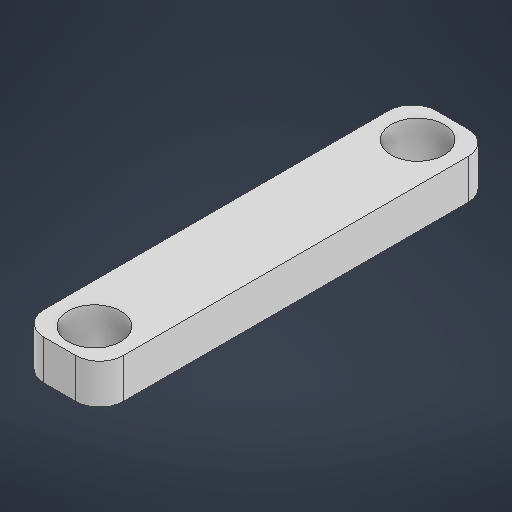
# Autodesk Inventor part: LegLverr
Saved by Autodesk Inventor 2026.2 (Build 302298010, 298A)
## iProperties
Created: 2026-05-06
Part Number: LegLverr
Material: Generic
Document SubType Name: Modeling
Designer: Martina
Density: 1 g/cm^3
Appearance: Default
Author: Martina
Autodesk Inventor part; units mm, degrees
ref_plane "YZ Plane" through (0, 0, 0) normal (1, 0, 0) x (0, 1, 0)
ref_plane "XZ Plane" through (0, 0, 0) normal (0, 1, 0) x (-1, 0, 0)
ref_plane "XY Plane" through (0, 0, 0) normal (0, 0, 1) x (1, 0, 0)
sketch "Sketch1" plane through (0, 0, 0) normal (0, 1, 0) x (-1, 0, 0)
  line L0 (3.6, 44.409) -> (-3.6, 44.409)
  line L1 (-9, 39.009) -> (-9, -39.009)
  line L2 (-3.6, -44.409) -> (3.6, -44.409)
  line L3 (9, -39.009) -> (9, 39.009)
  line L4 (9, 44.409) -> (-9, -44.409) construction
  line L5 (-9, 44.409) -> (9, -44.409) construction
  arc A0 (3.6, -44.409) -> (9, -39.009) centre (3.6, -39.009) ccw
  arc A1 (-9, -39.009) -> (-3.6, -44.409) centre (-3.6, -39.009) ccw
  arc A2 (9, 39.009) -> (3.6, 44.409) centre (3.6, 39.009) ccw
  arc A3 (-3.6, 44.409) -> (-9, 39.009) centre (-3.6, 39.009) ccw
  line L6 (0, -44.409) -> (0, -36.591)
  circle A4 centre (0, -36.591) radius 6
  line L7 (0, 0) -> (1.5436, 0)
  circle A5 centre (0, 36.591) radius 6
  dimension "d0" = 18
  dimension "d1" = 88.818
  dimension "d2" = 5.4
  dimension "d3" = 7.818
  dimension "d4" = 12
  constraints: 16 end point, 8 point on circle, 8 point on line, 8 tangent, 6 centre point, 3 equal radius, 3 midpoint, 2 horizontal, 2 parallel, 2 perpendicular, 1 coincident, 1 symmetric about line, 1 vertical, 1 other
  measures "d0" distance of L5.end L4.end
  measures "d1" distance of L4.end L5.start
  measures "d2" radius of A0
  measures "d3" distance of L6.start L6.end
  measures "d4" diameter of A4
extrude "Extrusion1" add sketch "Sketch1" along normal blind 9
body "Solid1"
